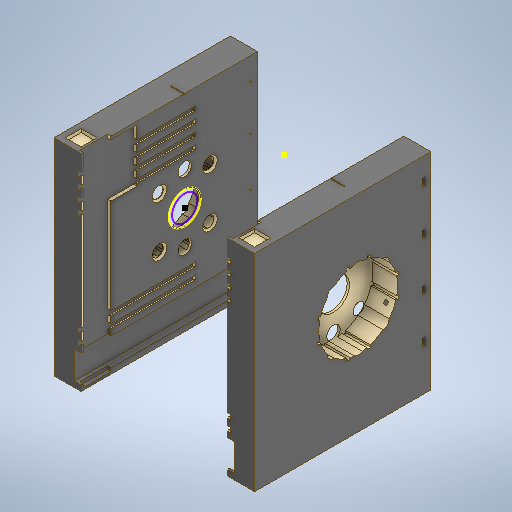
# Autodesk Inventor part: 2024_09_24_Reaktorkorpus_links+rechts
Saved by Autodesk Inventor 2025.1 (Build 291241000, 241)
## iProperties
Created: 2020-09-23
Part Number: 2024_09_24_Reaktorkorpus_links+rechts
Material: Acetalharz, Weiß
Document SubType Name: Modeling
Designer: Daniel
Density: 1.425 g/cm^3
Appearance: Beige
Author: Daniel
Autodesk Inventor part; units mm, degrees
(part 1 of 3)
ref_plane "YZ Plane" through (0, 0, 0) normal (1, 0, 0) x (0, 1, 0)
sketch "Skizze1" plane through (0, 0, 0) normal (0, 0, 1) x (1, 0, 0)
  line L0 (89, -91.5) -> (-89, -91.5)
  line L1 (-89, -91.5) -> (-89, 91.5)
  line L2 (-89, 91.5) -> (89, 91.5)
  line L3 (89, 91.5) -> (89, -91.5)
  line L4 (89, -91.5) -> (-89, 91.5) construction
  line L5 (-89, -91.5) -> (89, 91.5) construction
  point P0 (0, 0)
  dimension "d0" = 183
  dimension "d1" = 178
  constraints: 12 end point, 2 midpoint, 2 parallel, 1 horizontal, 1 perpendicular
  measures "d0" distance of L0.end L1.end
  measures "d1" distance of L1.end L2.end
extrude "Extrusion1" add sketch "Skizze1" along normal blind 24
sketch "Skizze2" plane through (0, 0, 24) normal (0, 0, 1) x (1, 0, 0)
  line L0 (-89, 91.5) -> (-89, -91.5) projected
  line L1 (-89, -91.5) -> (89, -91.5) projected
  line L2 (-89, 91.5) -> (89, 91.5)
  line L3 (89, 91.5) -> (89, -91.5)
  line L4 (89, -91.5) -> (-89, -91.5)
  line L5 (-89, -91.5) -> (-89, 91.5)
  line L6 (87, -89.5) -> (-87, -89.5)
  line L7 (-87, -89.5) -> (-87, 89.5)
  line L8 (-87, 89.5) -> (87, 89.5)
  line L9 (87, 89.5) -> (87, -89.5)
  line L10 (87, -89.5) -> (-87, 89.5) construction
  line L11 (-87, -89.5) -> (87, 89.5) construction
  line L12 (-70, -89.5) -> (70, -89.5)
  line L13 (70, -89.5) -> (70, 89.5)
  line L14 (70, 89.5) -> (-70, 89.5)
  line L15 (-70, 89.5) -> (-70, -89.5)
  line L16 (-70, -89.5) -> (70, 89.5) construction
  line L17 (70, -89.5) -> (-70, 89.5) construction
  line L18 (-65, -89.5) -> (65, -89.5)
  line L19 (65, -89.5) -> (65, 89.5)
  line L20 (65, 89.5) -> (-65, 89.5)
  line L21 (-65, 89.5) -> (-65, -89.5)
  line L22 (-65, -89.5) -> (65, 89.5) construction
  line L23 (65, -89.5) -> (-65, 89.5) construction
  line L24 (-65, 89.5) -> (-65, 91.5)
  line L25 (89, 91.5) -> (-89, 91.5) projected
  line L26 (-65, -89.5) -> (-65, -91.5)
  line L27 (65, -89.5) -> (65, -91.5)
  line L28 (65, 89.5) -> (65, 91.5)
  line L29 (89, -91.5) -> (89, 91.5) projected
  line L30 (-89, -91.5) -> (89, -91.5)
  line L31 (89, -91.5) -> (89, -86.5)
  line L32 (89, -86.5) -> (-89, -86.5)
  line L33 (-89, -86.5) -> (-89, -91.5)
  point P0 (0, 0)
  point P1 (70, -89.5)
  point P2 (87, -86.5)
  point P3 (70, -86.5)
  point P4 (-70, -86.5)
  point P5 (-87, -86.5)
  dimension "d4" = 2
  dimension "d5" = 2
  dimension "d6" = 17
  dimension "d7" = 24
  dimension "d10" = 5
  constraints: 60 end point, 11 parallel, 9 point on line, 6 midpoint, 6 perpendicular, 5 horizontal
  measures "d4" distance between parallel lines of L2 L8
  measures "d5" distance between parallel lines of L0 L7
  measures "d6" distance between parallel lines of L9 L13
  measures "d7" distance between parallel lines of L19 L3
  measures "d10" distance between parallel lines of L1 L32
extrude "Extrusion2" add sketch "Skizze2" along normal blind 156.5 contours L2 L24 L8 L7 L32 L0 | L32 L7 L6 L26 L1 L0 | L32 L15 L6 L7 | L2 L3 L32 L9 L8 L28 | L21 L32 L15 L8 | L32 L21 L6 L15 | L8 L13 L32 L19 | L27 L6 L9 L32 L3 L1 | L32 L13 L6 L19 | L9 L6 L13 L32
sketch "Skizze3" plane through (-89, 91.5, 0) normal (0, 1, 0) x (1, 0, 0)
  line L0 (0, 0) -> (0, -180.5) projected
  line L1 (0, -180.5) -> (55, -235.5)
  line L2 (0, -180.5) -> (24, -180.5) projected
  line L3 (24, -180.5) -> (-22.6667, -227.1667)
  line L4 (154, -24) -> (154, -180.5) projected
  line L5 (154, -180.5) -> (202, -228.5)
  line L6 (178, 0) -> (178, -180.5) projected
  line L7 (178, -180.5) -> (113.5, -245)
  line L8 (178, -180.5) -> (154, -180.5) projected
  line L9 (2, -24) -> (2, -180.5) projected
  line L10 (2, -180.5) -> (13, -191.5)
  line L11 (19, -180.5) -> (9.5, -190)
  line L12 (159, -24) -> (159, -180.5) projected
  line L13 (159, -180.5) -> (169, -189.5)
  line L14 (176, -24) -> (176, -180.5) projected
  line L15 (176, -180.5) -> (165, -191.5)
  point P0 (89, 0)
  point P1 (167.9474, -188.5526)
  point P2 (166, -192.5)
  point P3 (10.5, -189)
  point P4 (12, -192.5)
  dimension "d11" = 45
  dimension "d12" = 45
  dimension "d13" = 45
  dimension "d14" = 45
  constraints: 16 end point, 5 point on line, 3 perpendicular
  measures "d11" angle of L3 L2
  measures "d12" angle of L1 L2
  measures "d13" angle of L5 L8
  measures "d14" angle of L8 L7
extrude "Extrusion3" add sketch "Skizze3" against normal up to surface (183 mm away) contours L2 L10 L11 L1 | L11 L10 L3 L1 | L11 L2 L3 L10 | L8 L13 L15 L5 | L15 L13 L7 L5 | L15 L8 L7 L13
sketch "Skizze4" plane through (-89, -91.5, 0) normal (0, -1, 0) x (1, 0, 0)
  line L0 (19, 180.5) -> (10.5, 189) projected
  line L1 (10.5, 189) -> (19, 180.5)
  line L2 (2, 24) -> (2, 180.5) projected
  line L3 (19, 180.5) -> (2, 180.5)
  line L4 (10.5, 189) -> (2, 180.5) projected
  line L5 (2, 180.5) -> (10.5, 189)
  line L6 (167.9474, 188.5526) -> (159, 180.5) projected
  line L7 (176, 180.5) -> (167.9474, 188.5526) projected
  line L8 (159, 180.5) -> (167.9474, 188.5526)
  line L9 (159, 180.5) -> (176, 180.5) projected
  line L10 (167.9474, 188.5526) -> (176, 180.5)
  line L11 (176, 180.5) -> (159, 180.5)
  point P0 (89, 0)
  constraints: 12 end point, 2 collinear, 1 horizontal, 1 perpendicular
extrude "Extrusion4" add sketch "Skizze4" against normal blind 5
sketch "Skizze5" plane through (-89, 91.5, 0) normal (0, 1, 0) x (1, 0, 0)
  line L0 (10.5, -189) -> (2, -180.5) projected
  line L1 (2, -180.5) -> (10.5, -189)
  line L2 (10.5, -189) -> (19, -180.5)
  line L3 (19, -180.5) -> (10.5, -189) projected
  line L4 (2, -180.5) -> (19, -180.5)
  line L5 (167.9474, -188.5526) -> (159, -180.5) projected
  line L6 (176, -180.5) -> (167.9474, -188.5526) projected
  line L7 (159, -180.5) -> (176, -180.5)
  line L8 (159, -180.5) -> (167.9474, -188.5526)
  line L9 (176, -180.5) -> (167.9474, -188.5526)
  point P0 (89, 0)
  constraints: 13 end point, 3 collinear, 2 horizontal
extrude "Extrusion5" add sketch "Skizze5" against normal blind 2
sketch "Skizze6" plane through (0, 0, 0) normal (0, 0, -1) x (-1, 0, 0)
  line L0 (89, 91.5) -> (89, -91.5) projected
  line L1 (-89, -91.5) -> (89, -91.5)
  line L2 (89, -91.5) -> (89, -86.5)
  line L3 (89, -86.5) -> (-89, -86.5)
  line L4 (-89, -86.5) -> (-89, -91.5)
  line L5 (-89, -86.5) -> (89, -86.5)
  line L6 (89, -86.5) -> (89, -62.5)
  line L7 (89, -62.5) -> (-89, -62.5)
  line L8 (-89, -62.5) -> (-89, -86.5)
  line L9 (-89, -91.5) -> (-89, 91.5) projected
  line L10 (-89, 91.5) -> (89, 91.5)
  line L11 (89, 91.5) -> (89, 67.5)
  line L12 (89, 67.5) -> (-89, 67.5)
  line L13 (-89, 67.5) -> (-89, 91.5)
  line L14 (-89, 67.5) -> (89, -62.5) construction
  line L15 (89, 67.5) -> (-89, -62.5) construction
  line L16 (-75.35, -64) -> (75.35, -64)
  line L17 (75.35, -64) -> (75.35, 69)
  line L18 (75.35, 69) -> (-75.35, 69)
  line L19 (-75.35, 69) -> (-75.35, -64)
  line L20 (-75.35, -64) -> (75.35, 69) construction
  line L21 (75.35, -64) -> (-75.35, 69) construction
  point P0 (0, 0)
  point P1 (0, 2.5)
  dimension "d21" = 5
  dimension "d22" = 24
  dimension "d23" = 24
  dimension "d24" = 150.7
  dimension "d25" = 133
  constraints: 40 end point, 8 parallel, 4 horizontal, 4 perpendicular, 3 midpoint, 3 point on line
  measures "d21" distance between parallel lines of L1 L3
  measures "d22" distance between parallel lines of L3 L7
  measures "d23" distance between parallel lines of L12 L10
  measures "d24" distance of L17.end L18.end
  measures "d25" distance of L18.end L16.start
extrude "Extrusion6" cut sketch "Skizze6" against normal blind 3 contours L17 L7 L19 L12 | L12 L19 L18 L17 | L17 L16 L19 L7
sketch "Skizze7" plane through (0, 0, 3) normal (0, 0, -1) x (-1, 0, 0)
  line L0 (-75.35, 69) -> (75.35, -64) construction
  line L1 (75.35, -64) -> (75.35, 69) construction
  line L2 (75.35, 69) -> (-75.35, -64) construction
  line L3 (-55.1, 48.75) -> (55.1, 48.75)
  line L4 (55.1, 48.75) -> (55.1, -43.75)
  line L5 (55.1, -43.75) -> (-55.1, -43.75)
  line L6 (-55.1, -43.75) -> (-55.1, 48.75)
  line L7 (-55.1, 48.75) -> (55.1, -43.75) construction
  line L8 (55.1, 48.75) -> (-55.1, -43.75) construction
  line L9 (-75.35, 69) -> (75.35, 69) projected
  line L10 (75.35, -64) -> (-75.35, -64) projected
  line L11 (0, 2.5) -> (75.35, 2.5) construction
  line L12 (-75.35, -64) -> (-75.35, 69) projected
  line L13 (0, 2.5) -> (-75.35, 2.5) construction
  line L14 (-60.35, -49) -> (-60.35, 55.7618) construction
  line L15 (0, -49) -> (-60.35, -49) construction
  line L16 (0, -49) -> (60.35, -49) construction
  line L17 (60.35, -49) -> (60.35, 2.5) construction
  line L18 (60.35, 2.5) -> (60.35, 54) construction
  line L19 (60.35, 54) -> (0, 54) construction
  line L20 (0, 54) -> (60.35, 54) construction
  circle A0 centre (0, 54) radius 1.7
  circle A1 centre (60.35, 54) radius 1.7
  circle A2 centre (60.35, 2.5) radius 1.7
  circle A3 centre (60.35, -49) radius 1.7
  circle A4 centre (0, -49) radius 1.7
  circle A5 centre (-60.35, -49) radius 1.7
  circle A6 centre (-60.35, 2.5) radius 1.7
  line L21 (0, 54) -> (-60.35, 54) construction
  circle A7 centre (-60.35, 54) radius 1.7
  point P0 (-60.35, 2.5)
  point P1 (60.35, 2.5)
  point P2 (0, 0)
  dimension "d105" = 92.5
  dimension "d106" = 110.2
  dimension "d107" = 15
  dimension "d108" = 15
  dimension "d109" = 15
  dimension "d110" = 15
  dimension "d112" = 3.4
  dimension "d113" = 3.4
  dimension "d114" = 3.4
  dimension "d115" = 3.4
  dimension "d116" = 3.4
  dimension "d117" = 3.4
  dimension "d118" = 3.4
  dimension "d119" = 0
  dimension "d120" = 0
  dimension "d121" = 0
  dimension "d122" = 0
  dimension "d123" = 0
  dimension "d125" = 0
  dimension "d126" = 0
  dimension "d127" = 0
  dimension "d128" = 0
  dimension "d129" = 0
  dimension "d130" = 0
  dimension "d131" = 3.4
  dimension "d132" = 120.7
  dimension "d133" = 103
  dimension "d134" = 2.5
  constraints: 38 end point, 8 centre point, 7 point on line, 5 midpoint, 4 perpendicular, 2 horizontal, 2 parallel, 2 vertical
  measures "d105" distance of L5.end L3.start
  measures "d106" distance of L3.start L3.end
  measures "d107" distance from line of L9 L19.end
  measures "d108" distance from line of L10 L15.start
  measures "d109" distance from line of L17.end L1
  measures "d110" distance from line of L12 point (-60.35, 2.5)
  measures "d112" diameter of A0
  measures "d113" diameter of A1
  measures "d114" diameter of A2
  measures "d115" diameter of A3
  measures "d116" diameter of A4
  measures "d117" diameter of A5
  measures "d118" diameter of A6
  measures "d119" distance of L21.start L19.end
  measures "d120" distance of point (-60.35, 2.5) A6.centre
  measures "d121" distance of A4.centre L15.start
  measures "d122" distance of L17.end A2.centre
  measures "d123" distance from line of A6.centre L14
  measures "d125" distance of A5.centre L14.start
  measures "d126" distance of A5.centre L14.start
  measures "d127" distance of A3.centre L16.end
  measures "d128" distance of L16.end A3.centre
  measures "d129" distance of L18.end A1.centre
  measures "d130" distance of L18.end A1.centre
  measures "d131" diameter of A7
  measures "d132" distance of A2.centre A6.centre
  measures "d133" distance of A4.centre L21.start
  measures "d134" distance of point (0, 0) L11.start
extrude "Extrusion7" cut sketch "Skizze7" against normal through all
sketch "Skizze8" plane through (-89, -91.5, 0) normal (0, -1, 0) x (1, 0, 0)
  line L0 (0, 0) -> (0, 180.5) projected
  line L1 (24, 24) -> (24, 180.5) projected
  line L2 (0, 180.5) -> (24, 180.5)
  line L3 (24, 180.5) -> (24, 156.5)
  line L4 (24, 156.5) -> (0, 156.5)
  line L5 (0, 156.5) -> (0, 180.5)
  line L6 (154, 24) -> (154, 180.5) projected
  line L7 (178, 0) -> (178, 180.5) projected
  line L8 (154, 180.5) -> (178, 180.5)
  line L9 (178, 180.5) -> (178, 156.5)
  line L10 (178, 156.5) -> (154, 156.5)
  line L11 (154, 156.5) -> (154, 180.5)
  line L12 (178, 0) -> (0, 0) projected
  line L13 (178, 0) -> (154, 0)
  line L14 (154, 0) -> (154, 24)
  line L15 (154, 24) -> (178, 24)
  line L16 (178, 24) -> (178, 0)
  line L17 (0, 0) -> (24, 0)
  line L18 (24, 0) -> (24, 24)
  line L19 (24, 24) -> (0, 24)
  line L20 (0, 24) -> (0, 0)
  line L21 (0, 180.5) -> (24, 156.5) construction
  line L22 (24, 180.5) -> (0, 156.5) construction
  line L23 (154, 180.5) -> (178, 156.5) construction
  line L24 (178, 180.5) -> (154, 156.5) construction
  line L25 (154, 24) -> (178, 0) construction
  line L26 (178, 24) -> (154, 0) construction
  line L27 (0, 24) -> (24, 0) construction
  line L28 (24, 24) -> (0, 0) construction
  line L29 (5, 5) -> (19, 5)
  line L30 (19, 5) -> (19, 19)
  line L31 (19, 19) -> (5, 19)
  line L32 (5, 19) -> (5, 5)
  line L33 (5, 5) -> (19, 19) construction
  line L34 (19, 5) -> (5, 19) construction
  line L35 (159, 19) -> (173, 19)
  line L36 (173, 19) -> (173, 5)
  line L37 (173, 5) -> (159, 5)
  line L38 (159, 5) -> (159, 19)
  line L39 (159, 19) -> (173, 5) construction
  line L40 (173, 19) -> (159, 5) construction
  line L41 (159, 175.5) -> (173, 175.5)
  line L42 (173, 175.5) -> (173, 161.5)
  line L43 (173, 161.5) -> (159, 161.5)
  line L44 (159, 161.5) -> (159, 175.5)
  line L45 (159, 175.5) -> (173, 161.5) construction
  line L46 (173, 175.5) -> (159, 161.5) construction
  line L47 (5, 175.5) -> (19, 175.5)
  line L48 (19, 175.5) -> (19, 161.5)
  line L49 (19, 161.5) -> (5, 161.5)
  line L50 (5, 161.5) -> (5, 175.5)
  line L51 (5, 175.5) -> (19, 161.5) construction
  line L52 (19, 175.5) -> (5, 161.5) construction
  point P0 (89, 0)
  point P1 (12, 12)
  point P2 (166, 12)
  point P3 (166, 168.5)
  point P4 (12, 168.5)
  dimension "d38" = 24
  dimension "d39" = 24
  dimension "d40" = 14
  dimension "d41" = 14
  dimension "d187" = 14
  constraints: 96 end point, 16 parallel, 13 midpoint, 11 perpendicular, 10 point on line, 8 horizontal
  measures "d38" distance of L0.end L2.end
  measures "d39" distance between parallel lines of L4 L2
  measures "d40" distance of L47.start L47.end
  measures "d41" distance of L42.end L43.end
  measures "d187" distance of L35.start L35.end
extrude "Extrusion8" cut sketch "Skizze8" against normal blind 3 contours L32 L31 L30 L29 | L35 L36 L37 L38 | L41 L42 L43 L44 | L47 L48 L49 L50
ref_plane "Arbeitsebene1" through (77, 91.5, 192.5) normal (0, 0, -1) x (0, -1, 0)
sketch "Skizze9" plane through (77, 91.5, 192.5) normal (0, 0, -1) x (0, -1, 0)
  line L0 (183, -12) -> (0, -12) projected
  line L1 (183, 166) -> (178, 166)
  line L2 (178, 166) -> (178, -12)
  line L3 (178, -12) -> (183, -12)
  line L4 (183, -12) -> (183, 166)
  line L5 (183, 166) -> (183, -12) construction
  line L6 (183, 166) -> (178, -12) construction
  line L7 (183, -12) -> (178, 166) construction
  line L8 (180.5, 77) -> (134.2573, 77) construction
  line L9 (134.2573, 24.15) -> (134.2573, 129.85) construction
  line L10 (190.25, 79) -> (165.75, 79)
  line L11 (165.75, 79) -> (165.75, 75)
  line L12 (165.75, 75) -> (190.25, 75)
  line L13 (190.25, 75) -> (190.25, 79)
  line L14 (190.25, 79) -> (165.75, 75) construction
  line L15 (165.75, 79) -> (190.25, 75) construction
  line L16 (153.5, 148) -> (178, 148)
  line L17 (178, 148) -> (178, 6)
  line L18 (178, 6) -> (153.5, 6)
  line L19 (153.5, 6) -> (153.5, 148)
  line L20 (153.5, 148) -> (178, 6) construction
  line L21 (178, 148) -> (153.5, 6) construction
  line L22 (183, 142) -> (0, 142) projected
  line L23 (0, 12) -> (183, 12) projected
  point P0 (91.5, 77)
  point P1 (178, 77)
  point P2 (165.75, 77)
  point P3 (178, 148)
  dimension "d44" = 5
  dimension "d45" = 24.5
  dimension "d46" = 6
  dimension "d47" = 6
  constraints: 38 end point, 8 midpoint, 6 parallel, 3 horizontal, 3 perpendicular, 3 point on line
  measures "d44" distance between parallel lines of L4 L2
  measures "d45" distance of L11.end L12.end
  measures "d46" distance between parallel lines of L16 L22
  measures "d47" distance between parallel lines of L23 L18
extrude "Extrusion9" cut sketch "Skizze9" along normal up to surface (168.5 mm away) contours L18 L19 L23 L2 | L23 L19 L22 L2 L10 L11 L12 | L12 L11 L10 L2 | L19 L16 L2 L22
sketch "Skizze10" plane through (0, 0, 24) normal (0, 0, 1) x (1, 0, 0)
  line L0 (-71, -86.5) -> (-71, -62) construction
  line L1 (78.9474, -86.5) -> (71, -86.5) construction
  line L2 (-71, -62) -> (71, -86.5) construction
  line L3 (70, -62) -> (70, 89.5) construction
  line L4 (71, -86.5) -> (71, -61.9796) construction
  line L5 (71, -61.9796) -> (-71, -86.5) construction
  line L6 (-65, -86.5) -> (-87, -86.5) projected
  line L7 (-73.9133, -86.5) -> (-73.9133, -62)
  line L8 (-77, 91.5) -> (-77, -91.5) projected
  line L9 (-71, -62) -> (-65, -62) projected
  line L10 (-71, -62) -> (71, -62)
  line L11 (71, -62) -> (71, -86.5)
  line L12 (71, -86.5) -> (-71, -86.5)
  line L13 (-71, -86.5) -> (-71, -62)
  point P0 (0, 0)
  point P1 (0, -74.2398)
  constraints: 16 end point, 4 parallel, 1 horizontal, 1 midpoint, 1 perpendicular, 1 point on line
extrude "Extrusion10" cut sketch "Skizze10" against normal blind 3
sketch "Skizze11" plane through (-89, 91.5, 0) normal (0, 1, 0) x (1, 0, 0)
  line L0 (0, -180.5) -> (12, -192.5) projected
  line L1 (178, 0) -> (178, -180.5) projected
  line L2 (0, -180.5) -> (178, -180.5)
  line L3 (178, -180.5) -> (178, -178.5)
  line L4 (178, -178.5) -> (0, -178.5)
  line L5 (0, -178.5) -> (0, -180.5)
  line L6 (0, -180.5) -> (178, -178.5) construction
  line L7 (178, -180.5) -> (0, -178.5) construction
  line L8 (89, -179.5) -> (89, -173) construction
  line L9 (79, -190.75) -> (99, -190.75) construction
  line L10 (99, -190.75) -> (99, -166.25) construction
  line L11 (99, -166.25) -> (79, -166.25) construction
  line L12 (79, -166.25) -> (79, -190.75) construction
  line L13 (79, -190.75) -> (99, -166.25) construction
  line L14 (99, -190.75) -> (79, -166.25) construction
  line L15 (21, -154) -> (157, -154)
  line L16 (157, -154) -> (157, -178.5)
  line L17 (157, -178.5) -> (21, -178.5)
  line L18 (21, -178.5) -> (21, -154)
  line L19 (21, -154) -> (157, -178.5) construction
  line L20 (157, -154) -> (21, -178.5) construction
  line L21 (154, -24) -> (154, -180.5) projected
  line L22 (24, -24) -> (24, -180.5) projected
  point P0 (89, 0)
  point P1 (89, -178.5)
  point P2 (89, -166.25)
  point P3 (21, -178.5)
  dimension "d52" = 2
  dimension "d53" = 24.5
  dimension "d54" = 3
  dimension "d55" = 3
  constraints: 38 end point, 7 midpoint, 6 parallel, 3 horizontal, 3 perpendicular, 3 point on line, 1 vertical
  measures "d52" distance between parallel lines of L2 L4
  measures "d53" distance of L9.end L10.end
  measures "d54" distance between parallel lines of L16 L21
  measures "d55" distance between parallel lines of L18 L22
extrude "Extrusion11" cut sketch "Skizze11" against normal blind 181 contours L4 L21 L15 L16 | L4 L22 L15 L21 | L4 L18 L15 L22
sketch "Skizze12" plane through (77, 91.5, 192.5) normal (0, 0, -1) x (0, -1, 0)
  line L0 (178, 148) -> (153.5, 148) construction
  line L1 (153.5, 6) -> (178, 6) construction
  line L2 (153.5, 148) -> (178, 6) construction
  line L3 (178, 6) -> (153.5, 6) construction
  line L4 (153.5, 6) -> (178, 148) construction
  line L5 (165.75, 77) -> (145.75, 77) construction
  line L6 (145.75, 77) -> (145.75, 9) construction
  line L7 (0, 9) -> (153.5, 9) construction
  line L8 (145.75, 9) -> (145.75, 145) construction
  line L9 (0, 145) -> (153.5, 145) construction
  line L10 (135.75, 145) -> (135.75, 9) construction
  line L11 (135.75, 9) -> (125.75, 9) construction
  line L12 (125.75, 9) -> (125.75, 145) construction
  line L13 (115.75, 145) -> (115.75, 9) construction
  line L14 (115.75, 9) -> (105.75, 9) construction
  line L15 (105.75, 9) -> (105.75, 145) construction
  line L16 (95.75, 145) -> (95.75, 9) construction
  line L17 (95.75, 9) -> (85.75, 9) construction
  line L18 (85.75, 9) -> (85.75, 145) construction
  line L19 (75.75, 145) -> (75.75, 9) construction
  line L20 (75.75, 9) -> (65.75, 9) construction
  line L21 (65.75, 9) -> (65.75, 145) construction
  line L22 (55.75, 145) -> (55.75, 9) construction
  line L23 (45.75, 145) -> (45.75, 9) construction
  line L24 (35.75, 9) -> (35.75, 145) construction
  line L25 (25.75, 145) -> (25.75, 9) construction
  line L26 (15.75, 9) -> (15.75, 145) construction
  line L27 (153.5, 142) -> (0, 142) projected
  line L28 (0, 12) -> (153.5, 12) projected
  line L29 (149.75, 15) -> (141.75, 15)
  line L30 (141.75, 15) -> (141.75, 9)
  line L31 (141.75, 9) -> (149.75, 9)
  line L32 (149.75, 9) -> (149.75, 15)
  line L33 (149.75, 15) -> (141.75, 9) construction
  line L34 (141.75, 15) -> (149.75, 9) construction
  line L35 (149.75, 9) -> (147.75, 12)
  line L36 (141.75, 9) -> (143.75, 12)
  line L37 (143.75, 12) -> (147.75, 12)
  line L38 (133.75, 142) -> (137.75, 142)
  line L39 (131.75, 9) -> (139.75, 9)
  line L40 (139.75, 9) -> (137.75, 12)
  line L41 (131.75, 9) -> (133.75, 12)
  line L42 (133.75, 12) -> (137.75, 12)
  line L43 (123.75, 142) -> (127.75, 142)
  line L44 (121.75, 9) -> (129.75, 9)
  line L45 (129.75, 9) -> (127.75, 12)
  line L46 (121.75, 9) -> (123.75, 12)
  line L47 (123.75, 12) -> (127.75, 12)
  line L48 (113.75, 142) -> (117.75, 142)
  line L49 (111.75, 9) -> (119.75, 9)
  line L50 (119.75, 9) -> (117.75, 12)
  line L51 (111.75, 9) -> (113.75, 12)
  line L52 (113.75, 12) -> (117.75, 12)
  line L53 (103.75, 142) -> (107.75, 142)
  line L54 (101.75, 9) -> (109.75, 9)
  line L55 (109.75, 9) -> (107.75, 12)
  line L56 (101.75, 9) -> (103.75, 12)
  line L57 (103.75, 12) -> (107.75, 12)
  line L58 (93.75, 142) -> (97.75, 142)
  line L59 (91.75, 9) -> (99.75, 9)
  line L60 (99.75, 9) -> (97.75, 12)
  line L61 (91.75, 9) -> (93.75, 12)
  line L62 (93.75, 12) -> (97.75, 12)
  line L63 (83.75, 142) -> (87.75, 142)
  line L64 (81.75, 9) -> (89.75, 9)
  line L65 (89.75, 9) -> (87.75, 12)
  line L66 (81.75, 9) -> (83.75, 12)
  line L67 (83.75, 12) -> (87.75, 12)
  line L68 (73.75, 142) -> (77.75, 142)
  line L69 (71.75, 9) -> (79.75, 9)
  line L70 (79.75, 9) -> (77.75, 12)
  line L71 (71.75, 9) -> (73.75, 12)
  line L72 (73.75, 12) -> (77.75, 12)
  line L73 (63.75, 142) -> (67.75, 142)
  line L74 (61.75, 9) -> (69.75, 9)
  line L75 (69.75, 9) -> (67.75, 12)
  line L76 (61.75, 9) -> (63.75, 12)
  line L77 (63.75, 12) -> (67.75, 12)
  line L78 (53.75, 142) -> (57.75, 142)
  line L79 (51.75, 9) -> (59.75, 9)
  line L80 (59.75, 9) -> (57.75, 12)
  line L81 (51.75, 9) -> (53.75, 12)
  line L82 (53.75, 12) -> (57.75, 12)
  line L83 (41.75, 9) -> (49.75, 9)
  line L84 (49.75, 9) -> (47.75, 12)
  line L85 (41.75, 9) -> (43.75, 12)
  line L86 (43.75, 12) -> (47.75, 12)
  line L87 (34.1029, 142) -> (38.1029, 142)
  line L88 (31.75, 9) -> (39.75, 9)
  line L89 (39.75, 9) -> (37.75, 12)
  line L90 (31.75, 9) -> (33.75, 12)
  line L91 (33.75, 12) -> (37.75, 12)
  line L92 (23.75, 142) -> (27.75, 142)
  line L93 (21.75, 9) -> (29.75, 9)
  line L94 (29.75, 9) -> (27.75, 12)
  line L95 (21.75, 9) -> (23.75, 12)
  line L96 (23.75, 12) -> (27.75, 12)
  line L97 (14.25, 145) -> (19.75, 145)
  line L98 (14.25, 145) -> (14.25, 142)
  line L99 (14.1846, 142) -> (18.1846, 142)
  line L100 (11.75, 9) -> (19.75, 9)
  line L101 (19.75, 9) -> (17.75, 12)
  line L102 (11.75, 9) -> (13.75, 12)
  line L103 (13.75, 12) -> (17.75, 12)
  line L104 (19.75, 145) -> (17.657, 141.5913)
  line L105 (19.75, 145) -> (23.75, 145) construction
  line L106 (24.25, 145) -> (24.25, 142)
  line L107 (24.1846, 142) -> (28.1846, 142)
  line L108 (24.25, 145) -> (29.75, 145)
  line L109 (29.75, 145) -> (27.657, 141.5913)
  line L110 (39.75, 145) -> (37.657, 141.5913)
  line L111 (34.25, 145) -> (39.75, 145)
  line L112 (34.25, 145) -> (34.25, 142)
  line L113 (44.1029, 142) -> (48.1029, 142)
  line L114 (44.25, 145) -> (49.75, 145)
  line L115 (44.25, 145) -> (44.25, 142)
  line L116 (49.75, 145) -> (47.657, 141.5913)
  line L117 (54.1029, 142) -> (58.1029, 142)
  line L118 (59.75, 145) -> (57.657, 141.5913)
  line L119 (54.25, 145) -> (59.75, 145)
  line L120 (54.25, 145) -> (54.25, 142)
  line L121 (64.1029, 142) -> (68.1029, 142)
  line L122 (69.75, 145) -> (67.657, 141.5913)
  line L123 (64.25, 145) -> (69.75, 145)
  line L124 (64.25, 145) -> (64.25, 142)
  line L125 (74.1029, 142) -> (78.1029, 142)
  line L126 (79.75, 145) -> (77.657, 141.5913)
  line L127 (74.25, 145) -> (79.75, 145)
  line L128 (74.25, 145) -> (74.25, 142)
  line L129 (84.1029, 142) -> (88.1029, 142)
  line L130 (89.75, 145) -> (87.657, 141.5913)
  line L131 (84.25, 145) -> (89.75, 145)
  line L132 (84.25, 145) -> (84.25, 142)
  line L133 (94.1029, 142) -> (98.1029, 142)
  line L134 (99.75, 145) -> (97.657, 141.5913)
  line L135 (94.25, 145) -> (99.75, 145)
  line L136 (94.25, 145) -> (94.25, 142)
  line L137 (104.1029, 142) -> (108.1029, 142)
  line L138 (109.75, 145) -> (107.657, 141.5913)
  line L139 (104.25, 145) -> (109.75, 145)
  line L140 (104.25, 145) -> (104.25, 142)
  line L141 (114.1029, 142) -> (118.1029, 142)
  line L142 (119.75, 145) -> (117.657, 141.5913)
  line L143 (114.25, 145) -> (119.75, 145)
  line L144 (114.25, 145) -> (114.25, 142)
  line L145 (124.1029, 142) -> (128.1029, 142)
  line L146 (129.75, 145) -> (127.657, 141.5913)
  line L147 (124.25, 145) -> (129.75, 145)
  line L148 (124.25, 145) -> (124.25, 142)
  line L149 (134.1029, 142) -> (138.1029, 142)
  line L150 (139.75, 145) -> (137.657, 141.5913)
  line L151 (134.25, 145) -> (139.75, 145)
  line L152 (134.25, 145) -> (134.25, 142)
  line L153 (143.75, 142) -> (147.75, 142)
  line L154 (144.25, 145) -> (144.25, 141.8382)
  line L155 (144.25, 145) -> (149.75, 145)
  line L156 (149.75, 145) -> (147.657, 141.5913)
  line L157 (144.0472, 141.8382) -> (148.0472, 141.8382)
  point P0 (91.5, 77)
  point P1 (145.75, 12)
  point P2 (135.75, 12)
  point P3 (125.75, 12)
  point P4 (115.75, 12)
  point P5 (105.75, 12)
  point P6 (95.75, 12)
  point P7 (85.75, 12)
  point P8 (75.75, 12)
  point P9 (65.75, 12)
  point P10 (55.75, 12)
  point P11 (45.75, 12)
  point P12 (35.75, 12)
  point P13 (25.75, 12)
  point P14 (15.75, 12)
  point P15 (135.75, 142)
  point P16 (125.75, 142)
  point P17 (115.75, 142)
  point P18 (105.75, 142)
  point P19 (95.75, 142)
  point P20 (85.75, 142)
  point P21 (75.75, 142)
  point P22 (65.75, 142)
  point P23 (55.75, 142)
  point P24 (45.75, 142)
  point P25 (35.75, 142)
  point P26 (25.75, 142)
  point P27 (15.75, 142)
  point P28 (125.75, 145)
  point P29 (115.75, 145)
  point P30 (105.75, 145)
  point P31 (95.75, 145)
  point P32 (85.75, 145)
  point P33 (75.75, 145)
  point P34 (65.75, 145)
  point P35 (35.75, 145)
  point P36 (25.75, 145)
  point P37 (15.75, 145)
  point P38 (14.25, 142)
  point P39 (17.75, 12)
  point P40 (13.75, 12)
  point P41 (27.75, 12)
  point P42 (23.75, 12)
  point P43 (37.75, 12)
  point P44 (33.75, 12)
  point P45 (43.75, 12)
  point P46 (57.75, 12)
  point P47 (53.75, 12)
  point P48 (63.75, 12)
  point P49 (87.75, 12)
  point P50 (97.75, 12)
  point P51 (93.75, 12)
  point P52 (107.75, 12)
  point P53 (103.75, 12)
  point P54 (113.75, 12)
  point P55 (127.75, 12)
  point P56 (123.75, 12)
  point P57 (137.75, 12)
  point P58 (23.75, 142)
  point P59 (133.75, 142)
  point P60 (14.25, 142)
  point P61 (17.908, 142)
  point P62 (25.75, 145)
  point P63 (25.75, 145)
  point P64 (24.25, 145)
  point P65 (24.25, 142)
  point P66 (27.908, 142)
  point P67 (35.75, 145)
  point P68 (44.25, 145)
  point P69 (44.25, 142)
  point P70 (47.908, 142)
  point P71 (34.25, 145)
  point P72 (34.25, 142)
  point P73 (37.908, 142)
  point P74 (65.75, 145)
  point P75 (75.75, 145)
  point P76 (85.75, 145)
  point P77 (95.75, 145)
  point P78 (105.75, 145)
  point P79 (115.75, 145)
  point P80 (125.75, 145)
  point P81 (134.25, 145)
  point P82 (137.908, 142)
  point P83 (144.25, 145)
  point P84 (144.25, 142.0022)
  point P85 (147.8087, 141.8382)
  dimension "d58" = 20
  dimension "d59" = 10
  dimension "d60" = 10
  dimension "d61" = 10
  dimension "d62" = 10
  dimension "d63" = 10
  dimension "d64" = 10
  dimension "d65" = 10
  dimension "d66" = 10
  dimension "d67" = 10
  dimension "d68" = 10
  dimension "d69" = 10
  dimension "d70" = 10
  dimension "d71" = 10
  dimension "d75" = 8
  dimension "d76" = 2
  dimension "d77" = 2
  dimension "d313" = 5.5
  dimension "d314" = 4
  dimension "d315" = 121.55
  dimension "d316" = 5.5
  dimension "d317" = 4
  dimension "d318" = 5.5
  dimension "d319" = 4
  dimension "d320" = 5.5
  dimension "d321" = 4
  dimension "d322" = 5.5
  dimension "d323" = 4
  dimension "d324" = 5.5
  dimension "d325" = 4
  dimension "d326" = 5.5
  dimension "d327" = 4
  dimension "d328" = 5.5
  dimension "d329" = 4
  dimension "d330" = 5.5
  dimension "d331" = 4
  dimension "d332" = 5.5
  dimension "d333" = 4
  dimension "d334" = 5.5
  dimension "d335" = 4
  dimension "d336" = 5.5
  dimension "d337" = 4
  dimension "d338" = 5.5
  dimension "d339" = 4
  dimension "d341" = 5.5
  dimension "d342" = 4
  constraints: 304 end point, 36 point on line, 6 perpendicular, 5 vertical, 4 horizontal, 3 midpoint, 3 parallel, 1 coincident, 1 collinear, 1 equal length, 32 other
  measures "d58" distance of L5.start L5.end
  measures "d59" distance between parallel lines of L10 L8
  measures "d60" distance between parallel lines of L12 L10
  measures "d61" distance between parallel lines of L13 L12
  measures "d62" distance between parallel lines of L13 L15
  measures "d63" distance between parallel lines of L15 L16
  measures "d64" distance between parallel lines of L18 L16
  measures "d65" distance between parallel lines of L18 L19
  measures "d66" distance between parallel lines of L19 L21
  measures "d67" distance between parallel lines of L21 L22
  measures "d68" distance between parallel lines of L23 L22
  measures "d69" distance between parallel lines of L24 L23
  measures "d70" distance between parallel lines of L25 L24
  measures "d71" distance between parallel lines of L26 L25
  measures "d75" distance of L29.start L29.end
  measures "d76" distance from line of L30 L36.end
  measures "d77" distance from line of L32 L35.end
  measures "d313" distance of L97.start L97.end
  measures "d314" distance of L97.end L104.end
  measures "d315" angle of L104 L105
  measures "d316" distance of L108.start L109.start
  measures "d317" distance of L109.start L109.end
  measures "d318" distance of L111.start L111.end
  measures "d319" distance of L111.end L110.end
  measures "d320" distance of L114.start L116.start
  measures "d321" distance of L116.start L116.end
  measures "d322" distance of L119.start L119.end
  measures "d323" distance of L119.end L118.end
  measures "d324" distance of L123.start L123.end
  measures "d325" distance of L123.end L122.end
  measures "d326" distance of L127.start L127.end
  measures "d327" distance of L127.end L126.end
  measures "d328" distance of L131.start L131.end
  measures "d329" distance of L131.end L130.end
  measures "d330" distance of L135.start L135.end
  measures "d331" distance of L135.end L134.end
  measures "d332" distance of L139.start L139.end
  measures "d333" distance of L139.end L138.end
  measures "d334" distance of L143.start L143.end
  measures "d335" distance of L143.end L142.end
  measures "d336" distance of L147.start L147.end
  measures "d337" distance of L147.end L146.end
  measures "d338" distance of L151.start L151.end
  measures "d339" distance of L151.end L150.end
  measures "d341" distance of L155.start L155.end
  measures "d342" distance of L155.end L156.end
extrude "Extrusion12" cut sketch "Skizze12" along normal blind 114 contours L27 L98 L97 L104 | L27 L106 L108 L109 | L27 L112 L111 L110 | L27 L115 L114 L116 | L27 L152 L151 L150 | L154 L155 L156 L27 | L27 L156 L157 L154 | L28 L40 L39 L41 | L28 L84 L83 L85 | L28 L89 L88 L90 | L28 L94 L93 L95 | L28 L101 L100 L102 | L28 L35 L31 L36
sketch "Skizze13" plane through (-89, 91.5, 0) normal (0, 1, 0) x (1, 0, 0)
  line L0 (0, 0) -> (0, -180.5) projected
  line L1 (178, 0) -> (178, -180.5) projected
  line L2 (0, 0) -> (178, 0)
  line L3 (178, 0) -> (178, -178)
  line L4 (178, -178) -> (0, -178)
  line L5 (0, -178) -> (0, 0)
  line L6 (166, -192.5) -> (178, -180.5) projected
  line L7 (178, -178) -> (166, -178)
  line L8 (166, -178) -> (166, -192.5)
  line L9 (166, -192.5) -> (178, -192.5)
  line L10 (178, -192.5) -> (178, -178)
  line L11 (178, 0) -> (178, -180.5) construction
  line L12 (0, -178) -> (178, 0) construction
  line L13 (178, 0) -> (0, 0) construction
  line L14 (178, 0) -> (0, 0) construction
  line L15 (0, 0) -> (178, -178) construction
  line L16 (166, -89.5) -> (12, -89.5)
  line L17 (12, -89.5) -> (12, -88.5)
  line L18 (12, -88.5) -> (166, -88.5)
  line L19 (166, -88.5) -> (166, -89.5)
  line L20 (166, -89.5) -> (12, -88.5) construction
  line L21 (12, -89.5) -> (166, -88.5) construction
  line L22 (88.5, -166) -> (89.5, -166)
  line L23 (89.5, -166) -> (89.5, -12)
  line L24 (89.5, -12) -> (88.5, -12)
  line L25 (88.5, -12) -> (88.5, -166)
  line L26 (88.5, -166) -> (89.5, -12) construction
  line L27 (89.5, -166) -> (88.5, -12) construction
  line L28 (24, -154) -> (24, -24) projected
  line L29 (154, -154) -> (24, -154)
  line L30 (24, -154) -> (24, -24)
  line L31 (24, -24) -> (154, -24)
  line L32 (154, -24) -> (154, -154)
  line L33 (154, -154) -> (24, -24) construction
  line L34 (24, -154) -> (154, -24) construction
  point P0 (89, 0)
  point P1 (89, -89)
  point P2 (88.5, -88.5)
  point P3 (88.5, -89.5)
  point P4 (89.5, -89.5)
  point P5 (89.5, -88.5)
  dimension "d80" = 178
  dimension "d81" = 14.5
  dimension "d82" = 1
  dimension "d83" = 1
  dimension "d84" = 154
  dimension "d85" = 154
  dimension "d90" = 130
  dimension "d91" = 130
  constraints: 58 end point, 11 equal length, 7 midpoint, 5 horizontal, 5 perpendicular, 1 point on line
  measures "d80" distance between parallel lines of L4 L2
  measures "d81" distance between parallel lines of L4 L9
  measures "d82" distance of L16.end L17.end
  measures "d83" distance of L23.end L24.end
  measures "d84" distance of L24.end L22.start
  measures "d85" distance of L17.end L18.end
  measures "d90" distance of L28.end L31.end
  measures "d91" distance of L29.end L28.end
extrude "Extrusion13" cut sketch "Skizze13" against normal blind 1 contours L16 L32 L18 L19 | L16 L23 L18 L32 | L23 L29 L25 L16 | L16 L25 L18 L23 | L16 L28 L18 L25 | L23 L22 L25 L29 | L18 L25 L31 L23 | L16 L17 L18 L28 | L31 L25 L24 L23